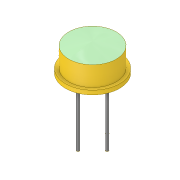
# Autodesk Inventor part: Photodiode
Saved by Autodesk Inventor 2017 (Build 210142000, 142)
## iProperties
Created: 2016-08-05
Part Number: Photodiode
Material: Generic
Document SubType Name: Modeling
Designer: ge937963
Density: 1 g/cm^3
Appearance: Glossy - Gold
Author: ge937963
Autodesk Inventor part; units mm, degrees
ref_plane "YZ Plane" through (0, 0, 0) normal (1, 0, 0) x (0, 1, 0)
ref_plane "XZ Plane" through (0, 0, 0) normal (0, 1, 0) x (-1, 0, 0)
ref_plane "XY Plane" through (0, 0, 0) normal (0, 0, 1) x (1, 0, 0)
sketch "Sketch1" plane through (0, 0, 0) normal (0, 0, 1) x (1, 0, 0)
  line L0 (0, 0) -> (0, 0.7112)
  line L1 (0, 0.7112) -> (3.81, 0.7112)
  line L2 (3.81, 0.7112) -> (3.81, 4.1402)
  line L3 (3.81, 4.1402) -> (4.1275, 4.1402)
  line L4 (4.1275, 4.1402) -> (4.1275, 0.7112)
  line L5 (4.1275, 0.7112) -> (4.699, 0.7112)
  line L6 (4.699, 0.7112) -> (4.699, 0)
  line L7 (4.699, 0) -> (0, 0)
  dimension "d0" = 0.7112
  dimension "d1" = 3.81
  dimension "d2" = 4.699
  dimension "d3" = 4.1275
  dimension "d4" = 4.1402
  constraints: 16 end point, 6 perpendicular, 2 point on line, 1 vertical
  measures "d0" distance of L0.start L0.end
  measures "d1" distance of L0.end L1.end
  measures "d2" distance from line of L0.start L6
  measures "d3" distance between parallel lines of L0 L4
  measures "d4" distance from line of L7 L2.end
revolve "Revolution1" add sketch "Sketch1" angle 360 about axis through (0, 0, 0) along (0, 1, 0)
sketch "Sketch2" plane through (0, 0, 0) normal (0, 0, 1) x (1, 0, 0)
  line L0 (-4.1275, 4.1402) -> (4.1275, 4.1402) projected
  line L1 (3.81, 0.7112) -> (3.81, 4.1402) projected
  line L2 (4.1275, 4.1402) -> (4.1275, 0.7112) projected
  line L3 (0, 4.1402) -> (0, 4.8253)
  arc A0 (4.1275, 4.1402) -> (0, 4.8253) centre (-0.4227, -10.4965) ccw
  arc A1 (3.81, 4.1402) -> (0, 4.5783) centre (-1.8241, -28.0728) ccw
  line L4 (-3.81, 4.1402) -> (3.81, 4.1402) projected
  line L5 (3.81, 4.1402) -> (4.1275, 4.1402)
  line L6 (0, 4.8253) -> (0, 4.5783)
  point P0 (0, 0)
  constraints: 6 end point, 4 point on circle, 2 centre point, 2 point on line, 1 collinear, 1 midpoint, 1 vertical
revolve "Revolution2" add sketch "Sketch2" angle 360 about axis through (0, 4.1402, 0) along (0, 1, 0) contours A1 L3 A0 L0
sketch "Sketch3" plane through (0, 0, 0) normal (0, -1, 0) x (1, 0, 0)
  line L0 (-4.4863, -0.3937) -> (-5.588, -0.3937)
  line L1 (-5.588, -0.3937) -> (-5.588, 0.3937)
  line L2 (-5.588, 0.3937) -> (-4.4863, 0.3937)
  line L3 (-4.4863, 0.3937) -> (-4.4863, -0.3937)
  circle A0 centre (0, 0) radius 4.699 projected
  point P0 (-5.588, 0)
  dimension "d7" = 0.7874
  dimension "d8" = 0.889
  constraints: 8 end point, 2 parallel, 1 horizontal, 1 horizontal alignment, 1 midpoint, 1 perpendicular
  measures "d7" distance of L0.end L1.end
  measures "d8" distance edge to line of A0 L1
extrude "Extrusion1" add sketch "Sketch3" against normal up to surface (0.7112 mm away) contours L0 A0 L2 L3 | L0 L1 L2 A0 picked at (-4.5566, -0.0438)
fillet "Fillet1" radius 0.1905 2 edges at (-5.588, 0.3556, -0.3937) (-5.588, 0.3556, 0.3937)
sketch "Sketch4" plane through (0, 0, 0) normal (0, -1, 0) x (1, 0, 0)
  circle A0 centre (0, 2.54) radius 0.2413
  circle A1 centre (-2.54, 0) radius 0.2413
  circle A2 centre (0, -2.54) radius 0.2413
  circle A3 centre (2.54, 0) radius 0.2413
  point P0 (0, 0)
  dimension "d12" = 0.4826
  dimension "d13" = 2.54
  dimension "d16" = 360
  constraints: 4 centre point, 9 other
  measures "d12" diameter of A0
  measures "d13" distance of A0.centre point (0, 0)
extrude "Extrusion2" add sketch "Sketch4" along normal blind 25.4
sketch "Sketch5" plane through (0, 0, 0) normal (0, 0, 1) x (1, 0, 0)
  line L0 (-8.3784, -29.1039) -> (8.218, -29.1039)
  line L1 (8.218, -29.1039) -> (8.218, -10.4229)
  line L2 (8.218, -10.4229) -> (-8.3784, -10.4229)
  line L3 (-8.3784, -10.4229) -> (-8.3784, -29.1039)
  point P0 (0, 0)
  constraints: 8 end point, 2 parallel, 1 horizontal, 1 perpendicular
extrude "Extrusion3" cut sketch "Sketch5" along normal through all both and the other way through all
body "Solid1"
